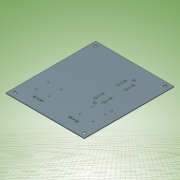
# Autodesk Inventor part: BaseProyecto
Saved by Autodesk Inventor 2022 (Build 260153000, 153)
## iProperties
Created: 2022-02-26
Part Number: BaseProyecto
Material: Genérico
Document SubType Name: Modeling
Designer: Marco
Density: 1 g/cm^3
Appearance: Valor por defecto
Author: Marco
Autodesk Inventor part; units mm, degrees
ref_plane "YZ Plane" through (0, 0, 0) normal (1, 0, 0) x (0, 1, 0)
ref_plane "XZ Plane" through (0, 0, 0) normal (0, 1, 0) x (-1, 0, 0)
ref_plane "XY Plane" through (0, 0, 0) normal (0, 0, 1) x (1, 0, 0)
sketch "Boceto1" plane through (0, 0, 0) normal (0, 1, 0) x (-1, 0, 0)
  line L0 (0, 0) -> (350, 0)
  line L1 (350, 0) -> (350, -400)
  line L2 (350, -400) -> (0, -400)
  line L3 (0, -400) -> (0, 0)
  circle A0 centre (20, -380) radius 6
  circle A1 centre (254.5115, -48) radius 2.5
  circle A2 centre (95.4885, -48) radius 2.5
  line L4 (245.5005, -51) -> (235.5005, -51)
  line L5 (235.5005, -51) -> (235.5005, -45)
  line L6 (235.5005, -45) -> (245.5005, -45)
  line L7 (245.5005, -45) -> (245.5005, -51)
  line L8 (273.5005, -51) -> (263.5005, -51)
  line L9 (263.5005, -51) -> (263.5005, -45)
  line L10 (263.5005, -45) -> (273.5005, -45)
  line L11 (273.5005, -45) -> (273.5005, -51)
  line L12 (114.4775, -51) -> (104.4775, -51)
  line L13 (104.4775, -51) -> (104.4775, -45)
  line L14 (104.4775, -45) -> (114.4775, -45)
  line L15 (114.4775, -45) -> (114.4775, -51)
  line L16 (86.4775, -51) -> (76.4775, -51)
  line L17 (76.4775, -51) -> (76.4775, -45)
  line L18 (76.4775, -45) -> (86.4775, -45)
  line L19 (86.4775, -45) -> (86.4775, -51)
  line L20 (254.5115, -48) -> (95.4885, -48) construction
  line L21 (114.4775, -45) -> (129.4775, -45) construction
  line L22 (129.4775, -45) -> (129.4775, -295) construction
  circle A3 centre (129.4775, -295) radius 2.5
  line L23 (132.4775, -315) -> (126.4775, -315)
  line L24 (126.4775, -315) -> (126.4775, -305)
  line L25 (126.4775, -305) -> (132.4775, -305)
  line L26 (132.4775, -305) -> (132.4775, -315)
  line L27 (132.4775, -285) -> (126.4775, -285)
  line L28 (126.4775, -285) -> (126.4775, -275)
  line L29 (126.4775, -275) -> (132.4775, -275)
  line L30 (132.4775, -275) -> (132.4775, -285)
  line L31 (132.4775, -215) -> (126.4775, -215)
  line L32 (126.4775, -215) -> (126.4775, -205)
  line L33 (126.4775, -205) -> (132.4775, -205)
  line L34 (132.4775, -205) -> (132.4775, -215)
  circle A4 centre (129.4775, -195) radius 2.5
  line L35 (132.4775, -185) -> (126.4775, -185)
  line L36 (126.4775, -185) -> (126.4775, -175)
  line L37 (126.4775, -175) -> (132.4775, -175)
  line L38 (132.4775, -175) -> (132.4775, -185)
  line L39 (96.4775, -315) -> (90.4775, -315)
  line L40 (90.4775, -315) -> (90.4775, -305)
  line L41 (90.4775, -305) -> (96.4775, -305)
  line L42 (96.4775, -305) -> (96.4775, -315)
  circle A5 centre (93.4775, -295) radius 2.5
  line L43 (96.4775, -285) -> (90.4775, -285)
  line L44 (90.4775, -285) -> (90.4775, -275)
  line L45 (90.4775, -275) -> (96.4775, -275)
  line L46 (96.4775, -275) -> (96.4775, -285)
  line L47 (96.4775, -215) -> (90.4775, -215)
  line L48 (90.4775, -215) -> (90.4775, -205)
  line L49 (90.4775, -205) -> (96.4775, -205)
  line L50 (96.4775, -205) -> (96.4775, -215)
  line L51 (96.4775, -185) -> (90.4775, -185)
  line L52 (90.4775, -185) -> (90.4775, -175)
  line L53 (90.4775, -175) -> (96.4775, -175)
  line L54 (96.4775, -175) -> (96.4775, -185)
  circle A6 centre (93.4775, -195) radius 2.5
  line L55 (116.4775, -335) -> (106.4775, -335)
  line L56 (106.4775, -335) -> (106.4775, -329)
  line L57 (106.4775, -329) -> (116.4775, -329)
  line L58 (116.4775, -329) -> (116.4775, -335)
  line L59 (116.4775, -161) -> (106.4775, -161)
  line L60 (106.4775, -161) -> (106.4775, -155)
  line L61 (106.4775, -155) -> (116.4775, -155)
  line L62 (116.4775, -155) -> (116.4775, -161)
  circle A7 centre (330, -380) radius 6
  circle A8 centre (330, -20) radius 6
  circle A9 centre (20, -20) radius 6
  line L63 (106.4775, -140) -> (41.4775, -140) construction
  line L64 (41.4775, -140) -> (41.4775, -80) construction
  line L65 (41.4775, -80) -> (106.4775, -80) construction
  line L66 (106.4775, -80) -> (106.4775, -140) construction
  circle A10 centre (42.4775, -166.3418) radius 2.5
  circle A11 centre (102.7945, -137.079) radius 2
  circle A12 centre (45.0335, -137.079) radius 2
  circle A13 centre (45.0335, -83.683) radius 2
  circle A14 centre (102.7945, -83.683) radius 2
  line L67 (301.4775, -140) -> (236.4775, -140) construction
  line L68 (236.4775, -140) -> (236.4775, -80) construction
  line L69 (236.4775, -80) -> (301.4775, -80) construction
  line L70 (301.4775, -80) -> (301.4775, -140) construction
  circle A15 centre (297.7945, -137.079) radius 2
  circle A16 centre (240.0335, -137.079) radius 2
  circle A17 centre (240.0335, -83.683) radius 2
  circle A18 centre (297.7945, -83.683) radius 2
  point P0 (235.5005, -48)
  point P1 (263.5005, -48)
  point P2 (104.4775, -48)
  point P3 (175, 0)
  point P4 (175, -48)
  point P5 (129.4775, -305)
  point P6 (129.4775, -285)
  point P7 (129.4775, -215)
  point P8 (129.4775, -275)
  point P9 (129.4775, -185)
  point P10 (126.4775, -310)
  point P11 (96.4775, -310)
  point P12 (93.4775, -305)
  point P13 (93.4775, -285)
  point P14 (93.4775, -215)
  point P15 (93.4775, -275)
  point P16 (93.4775, -205)
  point P17 (93.4775, -175)
  dimension "d0" = 350
  dimension "d1" = 400
  dimension "d4" = 12
  dimension "d5" = 20
  dimension "d6" = 20
  dimension "d7" = 5
  dimension "d8" = 5
  dimension "d11" = 10
  dimension "d12" = 6
  dimension "d13" = 10
  dimension "d15" = 18
  dimension "d16" = 6
  dimension "d17" = 9.011
  dimension "d18" = 10
  dimension "d19" = 6
  dimension "d20" = 10
  dimension "d21" = 6
  dimension "d22" = 18
  dimension "d23" = 9.011
  dimension "d26" = 121.023
  dimension "d27" = 45
  dimension "d29" = 15
  dimension "d30" = 250
  dimension "d31" = 5
  dimension "d33" = 10
  dimension "d34" = 6
  dimension "d35" = 10
  dimension "d36" = 20
  dimension "d37" = 10
  dimension "d39" = 10
  dimension "d40" = 60
  dimension "d41" = 6
  dimension "d42" = 5
  dimension "d43" = 10
  dimension "d44" = 6
  dimension "d45" = 10
  dimension "d46" = 20
  dimension "d48" = 10
  dimension "d50" = 42
  dimension "d51" = 6
  dimension "d52" = 6
  dimension "d53" = 5
  dimension "d54" = 6
  dimension "d55" = 10
  dimension "d56" = 5
  dimension "d57" = 20
  dimension "d58" = 10
  dimension "d59" = 6
  dimension "d60" = 10
  dimension "d61" = 10
  dimension "d62" = 6
  dimension "d64" = 16
  dimension "d66" = 10
  dimension "d67" = 6
  dimension "d68" = 16
  dimension "d70" = 20
  dimension "d71" = 20
  dimension "d73" = 20
  dimension "d77" = 20
  dimension "d81" = 65
  dimension "d82" = 60
  dimension "d83" = 5
  dimension "d84" = 11.3418
  dimension "d85" = 48
  constraints: 142 end point, 34 parallel, 19 centre point, 19 horizontal, 18 midpoint, 18 perpendicular, 12 vertical alignment, 11 horizontal alignment, 4 point on line, 3 equal radius, 1 coincident
  measures "d0" distance of L1.end L2.end
  measures "d1" distance of L0.end L1.end
  measures "d4" diameter of A0
  measures "d5" horizontal distance of L2.end A0.centre
  measures "d6" horizontal distance of A0.centre L2.end
  measures "d7" diameter of A1
  measures "d8" diameter of A2
  measures "d11" distance of L5.end L6.end
  measures "d12" distance of L4.end L5.end
  measures "d13" distance of L9.end L10.end
  measures "d15" distance of L9.end L6.end
  measures "d16" distance of L10.end L8.start
  measures "d17" horizontal distance of L4.start L20.start
  measures "d18" distance of L13.end L14.end
  measures "d19" distance of L12.end L13.end
  measures "d20" distance of L17.end L18.end
  measures "d21" distance of L16.end L17.end
  measures "d22" distance of L18.end L13.end
  measures "d23" horizontal distance of L16.start L20.end
  measures "d26" distance of L14.end L5.end
  measures "d27" vertical distance of L0.start L17.end
  measures "d29" distance of L14.end L21.end
  measures "d30" distance of L21.end L22.end
  measures "d31" diameter of A3
  measures "d33" distance of L23.end L24.end
  measures "d34" distance of L28.end L29.end
  measures "d35" distance of L27.end L28.end
  measures "d36" distance of L27.start L25.end
  measures "d37" vertical distance of L27.end A3.centre
  measures "d39" distance of L31.end L32.end
  measures "d40" distance of L31.end L28.end
  measures "d41" distance of L31.end L31.start
  measures "d42" diameter of A4
  measures "d43" vertical distance of A4.centre L32.end
  measures "d44" distance of L36.end L37.end
  measures "d45" distance of L35.end L36.end
  measures "d46" distance of L35.start L33.end
  measures "d48" distance of L39.end L40.end
  measures "d50" distance of L39.end L23.start
  measures "d51" distance of L39.end L39.start
  measures "d52" distance of L23.start L23.end
  measures "d53" diameter of A5
  measures "d54" distance of L44.end L45.end
  measures "d55" distance of L43.end L44.end
  measures "d56" diameter of A6
  measures "d57" distance of L51.end L48.end
  measures "d58" distance of L47.end L48.end
  measures "d59" distance of L47.start L47.end
  measures "d60" vertical distance of L51.start A6.centre
  measures "d61" distance of L56.end L57.end
  measures "d62" distance of L55.end L56.end
  measures "d64" horizontal distance of L39.end L55.end
  measures "d66" distance of L60.end L61.end
  measures "d67" distance of L59.end L60.end
  measures "d68" horizontal distance of L61.end L37.end
  measures "d70" vertical distance of L23.start L55.start
  measures "d71" vertical distance of L60.end L52.end
  measures "d73" horizontal distance of L1.end A7.centre
  measures "d77" horizontal distance of A8.centre L0.end
  measures "d81" distance of L64.end L65.end
  measures "d82" distance of L63.end L64.end
  measures "d83" diameter of A10
  measures "d84" vertical distance of L60.end A10.centre
  measures "d85" horizontal distance of A10.centre L52.end
extrude "Extrusión1" add sketch "Boceto1" along normal blind 3
